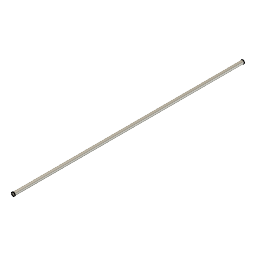
新轴心杆 (Autodesk Fusion 360 design; units mm, degrees)
part number: 2025-10-23-21-53-34-933
Autodesk Fusion 360 part; units mm, degrees
sketch "草图1" plane through (0, 0, 0) normal (1, 0, 0) x (0, 0, -1)
sketch "草图2" plane through (0, 0, 0) normal (0, 0, 1) x (1, 0, 0)
  circle A0 centre (0, 0) radius 1.4
  dimension "d2" = 2.8
  constraint coincident A0.centre origin
  measures "d2" diameter of A0
extrude "拉伸1" add sketch "草图2" along normal mid plane 160
extrude "拉伸2" add 1 faces at (0.5498, -0.3174, 80) along direction (0, 0, 1) blind 18
